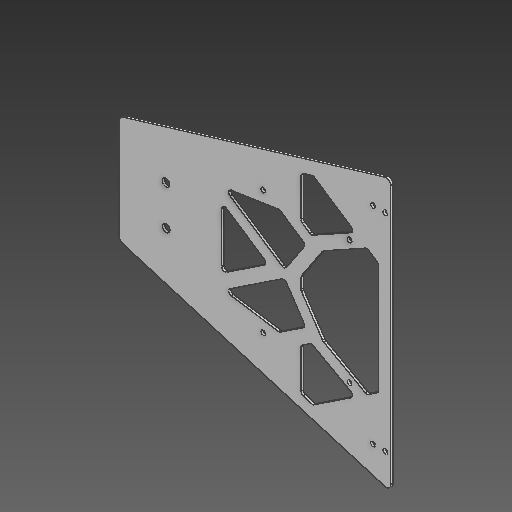
# Autodesk Inventor part: Part1
Saved by Autodesk Inventor 2025.2 (Build 292293000, 293)
## iProperties
Created: 2025-09-26
Part Number: Part1
Material: Generic
Document SubType Name: Sheet Metal
Designer: valer
Density: 1 g/cm^3
Sheet Metal Rule: Default
Appearance: Default
Author: valer
Autodesk Inventor part; units mm, degrees
ref_plane "YZ Plane" through (0, 0, 0) normal (1, 0, 0) x (0, 1, 0)
ref_plane "XZ Plane" through (0, 0, 0) normal (0, 1, 0) x (-1, 0, 0)
ref_plane "XY Plane" through (0, 0, 0) normal (0, 0, 1) x (1, 0, 0)
sketch "Base" plane through (0, 0, 0) normal (0, 0, 1) x (1, 0, 0)
  line L0 (-173.8499, -66.2658) -> (171.6188, -178.9186) construction
  line L1 (-9.525, -101.5493) -> (-9.525, 101.5493) construction
  line L2 (-9.525, 0) -> (-9.525, -119.85)
  line L3 (187.0398, -183.9472) -> (-9.525, -119.85)
  line L4 (187.0398, -183.9472) -> (187.0398, 0)
  line L5 (187.0398, 0) -> (-9.525, 0) construction
  line L6 (-9.525, 0) -> (-9.525, 119.85)
  line L7 (187.0398, 183.9472) -> (-9.525, 119.85)
  line L8 (187.0398, 183.9472) -> (187.0398, 0)
  point P0 (0, 0)
  point P1 (187.0398, -182.4643)
extrude "Plate1" add sketch "Base" along normal blind 3
sketch "MountHoles" plane through (0, 0, 0) normal (0, 0, -1) x (-1, 0, 0)
  line L0 (-179.0398, 172.9239) -> (1.525, 114.0441) construction
  circle A0 centre (-179.0398, 172.9239) radius 3
  circle A1 centre (1.525, 114.0441) radius 3
  line L1 (-226.3528, 0) -> (48.838, 0) construction
  circle A2 centre (-179.0398, -172.9239) radius 3
  circle A3 centre (1.525, -114.0441) radius 3
  line L2 (-187.0398, 183.9472) -> (9.525, 119.85) projected
  point P0 (0, 0)
  dimension "d2" = 6
  dimension "d3" = 6
  dimension "d45" = 8
  constraints: 4 centre point, 2 coincident, 2 end point, 2 symmetric about line, 2 other
  measures "d2" diameter of A0
  measures "d3" diameter of A1
  measures "d45" distance between parallel lines of L2 L0
extrude "MountHolesFeature" cut sketch "MountHoles" against normal blind 3
sketch "TorsoLiftMountHoles" plane through (0, 0, 3) normal (0, 0, 1) x (1, 0, 0)
  circle A0 centre (180.0398, -133.6037) radius 3 projected
  circle A1 centre (164.0398, -133.6037) radius 3 projected
  circle A2 centre (180.0398, 133.6037) radius 3 projected
  circle A3 centre (164.0398, 133.6037) radius 3 projected
  point P0 (0, 0)
extrude "TorsoLiftMountHolesFeature" cut sketch "TorsoLiftMountHoles" against normal blind 3
sketch "Continuation" plane through (0, 0, 0) normal (0, 0, -1) x (-1, 0, 0)
  line L0 (9.525, 119.85) -> (164.525, 69.3065)
  line L1 (-257.3528, 0) -> (234.838, 0) construction
  line L2 (9.525, -119.85) -> (164.525, -69.3065)
  line L3 (164.525, 69.3065) -> (164.525, -69.3065)
  line L4 (-187.0398, 183.9472) -> (9.525, 119.85)
  line L5 (9.525, 119.85) -> (9.525, -119.85)
  circle A0 centre (1.525, 114.0441) radius 3
  line L6 (1.525, 114.0441) -> (164.525, 60.8919) construction
  circle A1 centre (139.525, 69.0441) radius 3
  circle A2 centre (139.525, -69.0441) radius 3
  point P0 (0, 0)
  dimension "d46" = 155
  dimension "d47" = 25
  measures "d46" distance between parallel lines of L5 L3
  measures "d47" distance from line of L3 A1.centre
sheet face with bend "ContinuationFeature" sketch "Continuation" thickness 3 toward (0, 0, 1) bend radius 3 relief straight relief width 3 relief depth 1.5 contours L0 L3 L2 L5
bend "Bend2"
fillet "OutsideFilletsFeature" radius 8 4 edges at (187.0398, -183.9472, 1.5) (187.0398, 183.9472, 1.5) (-164.525, 69.3065, 1.5) (-164.525, -69.3065, 1.5)
ref_plane "MidPlane" through (0, -71.2585, 3.048) normal (1, 0, 0) x (0, 0, -1)
sketch "BottomMountHoles" plane through (0, 0, 0) normal (0, 0, -1) x (-1, 0, 0)
  circle A0 centre (18.4607, -50.75) radius 2.75 projected
  circle A1 centre (18.4607, -8.25) radius 2.75 projected
  circle A2 centre (18.4607, 8.25) radius 2.75 projected
  circle A3 centre (18.4607, 50.75) radius 2.75 projected
  ellipse E0 centre (103.3601, -25.3391) end of major axis (108.1225, -25.3596) minor radius 4.7625 projected
  ellipse E1 centre (103.5793, 25.4605) end of major axis (108.3417, 25.4399) minor radius 4.7625 projected
  spline S0 degree 3 poles (-22.2189, -83.25) (-22.5891, -83.25) (-22.9886, -83.178) (-23.6929, -82.9105) (-24.0824, -82.71) (-24.7238, -82.1045) (-24.9548, -81.7839) (-25.3958, -80.8943) (-25.4483, -80.428) (-25.4764, -79.9859) (-25.4838, -79.5156) (-25.1415, -78.5243) (-24.922, -78.15) (-24.3999, -77.5609) (-24.0923, -77.3244) (-23.5146, -77.014) (-23.2534, -76.9113) (-22.8383, -76.8067) (-22.5689, -76.75) (-22.2189, -76.75) knots 0 0 0 0 0.111053 0.111053 0.202489 0.202489 0.273701 0.273701 0.38581 0.38581 0.497395 0.497395 0.578796 0.578796 0.654724 0.654724 0.709985 0.709985 0.740525 0.740525 0.740525 0.740525 construction
  arc A4 (-22.2189, 83.25) -> (-22.2189, 76.75) centre (-22.2189, 80) ccw construction
  arc A5 (-133.7189, -83.25) -> (-133.7189, -76.75) centre (-133.7189, -80) ccw construction
  spline S1 degree 3 poles (-133.7189, 83.25) (-133.3487, 83.25) (-132.9492, 83.178) (-132.2449, 82.9105) (-131.8554, 82.71) (-131.2141, 82.1045) (-130.983, 81.7839) (-130.542, 80.8943) (-130.4896, 80.428) (-130.4615, 79.9859) (-130.4541, 79.5156) (-130.7963, 78.5243) (-131.0158, 78.15) (-131.538, 77.5609) (-131.8456, 77.3244) (-132.4232, 77.014) (-132.6845, 76.9113) (-133.0996, 76.8067) (-133.3689, 76.75) (-133.7189, 76.75) knots 0 0 0 0 0.111053 0.111053 0.202489 0.202489 0.273701 0.273701 0.38581 0.38581 0.497395 0.497395 0.578796 0.578796 0.654725 0.654725 0.709986 0.709986 0.740527 0.740527 0.740527 0.740527 construction
  line L0 (167.4427, 0) -> (-246.1203, 0) construction
  circle A6 centre (-133.7189, -80) radius 3
  circle A7 centre (-22.2189, 80) radius 3
  circle A8 centre (-22.2189, -80) radius 3
  circle A9 centre (-133.7189, 80) radius 3
  point P0 (0, 0)
  dimension "d80" = 6
  dimension "d81" = 6
  constraints: 4 centre point, 2 coincident, 2 symmetric about line, 2 other
  measures "d80" diameter of A6
  measures "d81" diameter of A7
extrude "Cut8" cut sketch "BottomMountHoles" against normal blind 3 contours E0 | E1 | A6 | A7 | A8 | A9
delete faces "Delete1" heal yes whole lump no faces at (-139.4042, 72.0417, 2) (-4.5153, 113.8027, 2) (179.1606, 175.9215, 2) (179.1606, -169.9264, 2) (-4.5153, -114.2855, 2) (-139.4042, -66.0465, 2)
sketch "Sketch15" plane through (187.0398, -172.9239, 3) normal (0, 0, 1) x (1, 0, 0)
  line L0 (-346.045, 244.0304) -> (-10.4802, 353.4537) projected
  line L1 (-346.045, 244.0304) -> (-0.3836, 348.2954)
  line L2 (-423.7471, 172.9239) -> (72.8866, 172.9239) construction
  line L3 (0, 345.8479) -> (0, 0) projected
  arc A0 (0, 345.8479) -> (-10.4802, 353.4537) centre (-8, 345.8479) ccw projected
  arc A1 (-346.045, 244.0304) -> (-351.5648, 236.4246) centre (-343.5648, 236.4246) ccw projected
  line L4 (-351.5648, 109.4233) -> (-351.5648, 236.4246) projected
  line L5 (-346.045, 101.8175) -> (-0.3836, -2.4475)
  arc A2 (-10.4802, -7.6058) -> (0, 0) centre (-8, 0) ccw projected
  line L6 (-10.4802, -7.6058) -> (-346.045, 101.8175) projected
  arc A3 (-351.5648, 109.4233) -> (-346.045, 101.8175) centre (-343.5648, 109.4233) ccw projected
  point P0 (-187.0398, 172.9239)
  dimension "d84" = 178.725
  constraints: 4 end point, 2 symmetric about line, 1 point on circle
  measures "d84" angle of L0 L1
extrude "AdjustToProductionFeature" cut sketch "Sketch15" against normal blind 3 contours L0 A0 L1 | L5 A2 L6
delete faces "Delete2" heal yes whole lump no faces at (187.0208, 173.4763, 1) (187.0208, -173.4763, 2)
fillet "Fillet5" radius 6 2 edges at (187.0398, 175.4872, 1.5) (187.0398, -175.4872, 1.5)
sketch "Sketch16" plane through (-164.525, -63.5006, 3) normal (0, 0, 1) x (1, 0, 0)
  line L0 (335.5648, 63.5006) -> (335.5648, -8.7511)
  line L1 (335.5648, -8.7511) -> (320.6792, -18.6535)
  line L2 (320.6792, -18.6535) -> (263.8755, 12.943)
  line L3 (263.8755, 12.943) -> (235.5648, 55.5006)
  line L4 (305.6902, -28.6247) -> (248.8865, 2.9718)
  line L5 (248.8865, 2.9718) -> (235.5648, -5.8901)
  line L6 (235.5648, -5.8901) -> (235.5648, -60.2844)
  line L7 (235.5648, -60.2844) -> (325.6009, -87.4427)
  line L8 (325.6009, -87.4427) -> (338.9225, -78.5808)
  line L9 (338.9225, -78.5808) -> (305.6902, -28.6247)
  line L10 (351.5648, -103.9097) -> (351.5648, 230.9109) construction
  line L11 (351.5648, 63.5006) -> (0, 63.5006) construction
  line L12 (0, 0) -> (0, 127.0012) projected
  line L13 (235.5648, 55.5006) -> (235.5648, 63.5006)
  line L14 (351.5648, 230.9109) -> (351.5648, -103.9097) projected
  line L15 (335.5648, 63.5006) -> (335.5648, 135.7524)
  line L16 (335.5648, 135.7524) -> (320.6792, 145.6548)
  line L17 (320.6792, 145.6548) -> (263.8755, 114.0583)
  line L18 (263.8755, 114.0583) -> (235.5648, 71.5006)
  line L19 (235.5648, 71.5006) -> (235.5648, 63.5006)
  line L20 (305.6902, -28.6247) -> (320.6792, -18.6535) construction
  line L21 (248.8865, 2.9718) -> (263.8755, 12.943) construction
  line L22 (5.5198, -7.6058) -> (343.8321, -109.654) construction
  line L23 (305.6902, 155.6259) -> (248.8865, 124.0294)
  line L24 (248.8865, 124.0294) -> (235.5648, 132.8914)
  line L25 (235.5648, 132.8914) -> (235.5648, 187.2856)
  line L26 (235.5648, 187.2856) -> (325.6009, 214.444)
  line L27 (325.6009, 214.444) -> (338.9225, 205.582)
  line L28 (338.9225, 205.582) -> (305.6902, 155.6259)
  line L29 (241.6919, 17.4027) -> (214.3249, 58.5418)
  line L30 (214.3249, 58.5418) -> (135.1659, 5.8828)
  line L31 (135.1659, 5.8828) -> (207.7779, -5.158)
  line L32 (207.7779, -5.158) -> (241.6919, 17.4027)
  line L33 (241.6919, 109.5986) -> (214.3249, 68.4595)
  line L34 (214.3249, 68.4595) -> (135.1659, 121.1185)
  line L35 (135.1659, 121.1185) -> (207.7779, 132.1593)
  line L36 (207.7779, 132.1593) -> (241.6919, 109.5986)
  line L37 (305.6902, -28.6247) -> (251.0683, -64.9608)
  line L38 (305.6902, 155.6259) -> (251.0683, 191.9621)
  point P0 (164.525, 63.5006)
  dimension "d88" = 16
  dimension "d89" = 16
  dimension "d90" = 16
  dimension "d91" = 16
  dimension "d92" = 16
  dimension "d93" = 16
  dimension "d94" = 16
  dimension "d95" = 16
  dimension "d96" = 60
  dimension "d97" = 65
  dimension "d98" = 100
  constraints: 70 end point, 15 symmetric about line, 9 parallel, 4 perpendicular, 3 point on line, 2 collinear, 2 midpoint, 1 vertical
  measures "d88" distance between parallel lines of L22 L7
  measures "d89" distance between parallel lines of L10 L0
  measures "d90" distance of L19.start L3.end
  measures "d91" distance of L4.end L5.end
  measures "d92" distance between parallel lines of L4 L2
  measures "d93" distance between parallel lines of L29 L3
  measures "d94" distance of L7.end L8.end
  measures "d95" distance between parallel lines of L32 L5
  measures "d96" distance of L8.end L4.start
  measures "d97" distance of L4.start L4.end
  measures "d98" distance between parallel lines of L13 L0
extrude "Cut10" cut sketch "Sketch16" against normal blind 3 contours L0 L1 L2 L3 L13 L19 L18 L17 L16 L15 | L37 L7 L6 L5 L4 | L23 L24 L25 L26 L38 | L32 L31 L30 L29 | L33 L34 L35 L36
fillet "Fillet6" radius 4 24 edges at (71.0398, -123.785, 1.5) (71.0398, -69.3908, 1.5) (84.3615, -60.5288, 1.5) (141.1652, -92.1253, 1.5) (156.1542, -82.1541, 1.5) (171.0398, -72.2518, 1.5) (99.3505, -50.5576, 1.5) (171.0398, 72.2518, 1.5) (156.1542, 82.1541, 1.5) (99.3505, 50.5576, 1.5) (71.0398, 8, 1.5) (71.0398, -8, 1.5) (141.1652, 92.1253, 1.5) (84.3615, 60.5288, 1.5) (71.0398, 69.3908, 1.5) (71.0398, 123.785, 1.5) (77.1669, -46.098, 1.5) (43.2529, -68.6586, 1.5) (-29.3591, -57.6178, 1.5) (49.7999, -4.9589, 1.5) (49.7999, 4.9589, 1.5) (77.1669, 46.098, 1.5) (43.2529, 68.6586, 1.5) (-29.3591, 57.6178, 1.5)
sketch "Sketch17" plane through (-164.525, -63.5006, 3) normal (0, 0, 1) x (1, 0, 0)
  line L0 (132.8917, 103.4145) -> (192.8917, 63.5006)
  line L1 (192.8917, 63.5006) -> (132.8917, 23.5868)
  line L2 (132.8917, 23.5868) -> (132.8917, 103.4145)
  line L3 (143.7792, 11.6126) -> (210.9945, 56.3263) projected
  line L4 (210.9945, 70.675) -> (143.7792, 115.3886) projected
  line L5 (0, 0) -> (0, 127.0012) projected
  point P0 (164.525, 63.5006)
  point P1 (132.8917, 63.5006)
  dimension "d102" = 16
  dimension "d103" = 16
  dimension "d104" = 60
  constraints: 6 end point, 3 parallel, 1 midpoint
  measures "d102" distance between parallel lines of L3 L1
  measures "d103" distance between parallel lines of L4 L0
  measures "d104" distance of point (132.892, 63.501) L0.end
extrude "Cut11" cut sketch "Sketch17" against normal blind 3
fillet "Fillet7" radius 4 3 edges at (28.3667, 0, 1.5) (-31.6333, 39.9139, 1.5) (-31.6333, -39.9139, 1.5)
equation "\"d7\" = Thickness"
equation "\"d43\" = Thickness"
equation "\"d82\" = Thickness"
equation "\"d85\" = Thickness"
equation "\"d99\" = Thickness"
equation "\"d0\" = Thickness"
equation "\"d48\" = BendRadius"
equation "\"d49\" = BendReliefWidth"
equation "\"d51\" = MinimumRemnant"
equation "\"d50\" = BendReliefDepth"
equation "\"d52\" = TransitionRadius"
equation "\"BendRadius\" = Thickness"
equation "\"BendReliefWidth\" = Thickness"
equation "\"BendReliefDepth\" = 0.5 * Thickness"
equation "\"CornerReliefSize\" = 4 * Thickness"
equation "\"MinimumRemnant\" = 2 * Thickness"
equation "\"TransitionRadius\" = BendRadius"
equation "\"JacobiRadiusSize\" = BendRadius"
equation "\"GapSize\" = Thickness"
equation "\"Thickness\" = 3"
body "Solid1"
